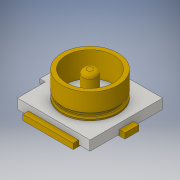
# Autodesk Inventor part: UMCC
Saved by Autodesk Inventor 2016 (Build 200138000, 138)
## iProperties
Created: 2016-08-30
Part Number: UMCC
Material: Generic
Document SubType Name: Modeling
Designer: jfixelle
Density: 1 g/cm^3
Appearance: Smooth - White
Author: jfixelle
Autodesk Inventor part; units mm, degrees
ref_plane "YZ Plane" through (0, 0, 0) normal (1, 0, 0) x (0, 1, 0)
ref_plane "XZ Plane" through (0, 0, 0) normal (0, 1, 0) x (-1, 0, 0)
ref_plane "XY Plane" through (0, 0, 0) normal (0, 0, 1) x (1, 0, 0)
sketch "Sketch1" plane through (0, 0, 0) normal (0, 1, 0) x (-1, 0, 0)
  line L0 (1.3, 1.3) -> (-1.3, 1.3)
  line L1 (-1.3, 1.3) -> (-1.3, -1.3)
  line L2 (-1.3, -1.3) -> (1.3, -1.3)
  line L3 (1.3, -1.3) -> (1.3, 1.3)
  line L4 (1.3, -0.872) -> (0.872, -1.3)
  point P0 (0, 0)
  dimension "d0" = 2.6
  dimension "d1" = 2.6
  dimension "d2" = 1.3
  dimension "d3" = 1.3
  dimension "d4" = 45
  constraints: 10 end point, 2 parallel, 2 point on line, 1 horizontal, 1 perpendicular
  measures "d0" distance of L2.end L0.start
  measures "d1" distance of L1.end L2.end
  measures "d2" distance from line of point (0, 0) L3
  measures "d3" distance from line of point (0, 0) L2
  measures "d4" angle of L3 L4
extrude "Extrusion1" add sketch "Sketch1" along normal blind 0.35 contours L3 L4 L2 L1 L0
sketch "Sketch2" plane through (0, 0, 0) normal (0, 1, 0) x (-1, 0, 0)
  line L0 (-0.9, 1.0436) -> (0.9, 1.0436)
  line L1 (0.9, 1.0436) -> (0.9, 1.5)
  line L2 (0.9, 1.5) -> (-0.9, 1.5)
  line L3 (-0.9, 1.5) -> (-0.9, 1.0436)
  line L4 (-0.9, -1.1545) -> (0.9, -1.1545)
  line L5 (0.9, -1.1545) -> (0.9, -1.5)
  line L6 (0.9, -1.5) -> (-0.9, -1.5)
  line L7 (-0.9, -1.5) -> (-0.9, -1.1545)
  line L8 (0.25, 0.25) -> (-1.5, 0.25)
  line L9 (-1.5, 0.25) -> (-1.5, -0.25)
  line L10 (-1.5, -0.25) -> (0.25, -0.25)
  line L11 (0.25, -0.25) -> (0.25, 0.25)
  line L12 (1.3, -0.872) -> (1.3, 1.3) projected
  point P0 (0, 0)
  dimension "d8" = 0.5
  dimension "d9" = 0.25
  dimension "d13" = 0.25
  dimension "d14" = 1.5
  dimension "d15" = 1.5
  dimension "d16" = 1.5
  dimension "d17" = 1.8
  dimension "d18" = 1.8
  dimension "d19" = 0.9
  dimension "d20" = 0.9
  constraints: 24 end point, 6 parallel, 3 horizontal, 3 perpendicular
  measures "d8" distance of L8.end L9.end
  measures "d9" distance from line of point (0, 0) L10
  measures "d13" distance from line of L11 point (0, 0)
  measures "d14" distance from line of point (0, 0) L9
  measures "d15" distance from line of L6 point (0, 0)
  measures "d16" distance from line of point (0, 0) L2
  measures "d17" distance of L1.end L2.end
  measures "d18" distance of L5.end L6.end
  measures "d19" distance from line of point (0, 0) L7
  measures "d20" distance from line of point (0, 0) L3
extrude "Extrusion2" add sketch "Sketch2" along normal blind 0.15 and the other way blind 0.05
sketch "Sketch3" plane through (0, 0.35, 0) normal (0, 1, 0) x (1, 0, 0)
  line L0 (-1.3, 0.872) -> (-1.3, -1.3) projected
  line L1 (-1.5, 0.3) -> (-1.3, 0.3)
  line L2 (-1.3, 0.3) -> (-1.3, -0.3)
  line L3 (-1.3, -0.3) -> (-1.5, -0.3)
  line L4 (-1.5, -0.3) -> (-1.5, 0.3)
  point P0 (0, 0)
  dimension "d25" = 1.5
  dimension "d26" = 0.6
  dimension "d27" = 0.3
  constraints: 8 end point, 2 parallel, 1 horizontal, 1 perpendicular, 1 point on line
  measures "d25" distance from line of L4 point (0, 0)
  measures "d26" distance of L3.end L1.start
  measures "d27" distance from line of point (0, 0) L1
extrude "Extrusion3" add sketch "Sketch3" against normal blind 0.15
sketch "Sketch4" plane through (0, 0.35, 0) normal (0, 1, 0) x (1, 0, 0)
  circle A0 centre (0, 0) radius 1
  circle A1 centre (0, 0) radius 0.25
  circle A2 centre (0, 0) radius 0.85
  dimension "d30" = 0.5
  dimension "d31" = 2
  dimension "d32" = 0.15
  constraints: 3 centre point, 3 coincident
  measures "d30" diameter of A1
  measures "d31" diameter of A0
  measures "d32" radial gap between concentric circles of A0 A2
extrude "Extrusion4" add sketch "Sketch4" along normal blind 0.9
fillet "Fillet1" radius 0.15 1 edges at (-0.25, 1.25, 0)
sketch "Sketch5" plane through (0, 0, 0) normal (1, 0, 0) x (0, 1, 0)
  line L0 (0.55, -1) -> (0.45, -1)
  line L1 (0.45, -1) -> (0.45, -0.9)
  line L2 (0.45, -0.9) -> (0.55, -0.9)
  line L3 (0.55, -0.9) -> (0.55, -1)
  line L4 (1.25, -1) -> (1.25, 1) projected
  line L5 (-0.31, 0) -> (1.51, 0) projected
  point P0 (0, 0)
  dimension "d36" = 0.1
  dimension "d37" = 0.7
  dimension "d38" = 1
  dimension "d39" = 0.1
  constraints: 8 end point, 2 parallel, 1 horizontal, 1 perpendicular
  measures "d36" distance of L0.start L0.end
  measures "d37" distance between parallel lines of L4 L3
  measures "d38" distance from line of point (0, 0) L0
  measures "d39" distance of L2.end L0.start
revolve "Revolution1" cut sketch "Sketch5" angle 360 about axis through (0, -10, 0) along (0, 1, 0)
chamfer "Chamfer1" distance 0.05 angle 45 1 edges at (-1, 0.45, 0)
chamfer "Chamfer2" distance 0.05 angle 45 1 edges at (-1, 0.55, 0)
body "Solid1"
